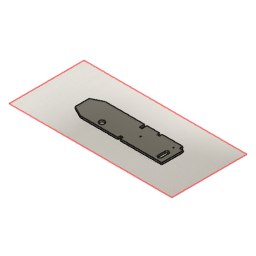
P_A22_ControlBoard v4 (Autodesk Fusion 360 design; units mm, degrees)
Autodesk Fusion 360 part; units mm, degrees
sketch "Sketch1" plane through (0, 0, 0) normal (0, 0, 1) x (1, 0, 0) in component "Component"
  line L0 (0, 23.2) -> (86.2, 23.2) construction
  line L1 (86.2, 23.2) -> (86.2, 0) construction
  line L2 (86.2, 0) -> (0, 0) construction
  line L3 (0, 0) -> (0, 23.2) construction
  line L4 (86.2, 20.3) -> (82.8, 20.3)
  line L5 (82.8, 20.3) -> (82.8, 23.2)
  line L6 (82.8, 23.2) -> (63.2045, 23.2)
  line L7 (63.3, 23.2) -> (63.3, 20.8)
  line L8 (63.3, 20.8) -> (61.1, 20.8)
  line L9 (61.1, 20.8) -> (61.1, 23.2)
  line L10 (61.1, 23.2) -> (49.1, 23.2)
  line L11 (49.1, 23.2) -> (49.1, 18.6)
  line L12 (49.1, 18.6) -> (46.9, 18.6)
  line L13 (46.9, 18.6) -> (46.9, 23.2)
  line L14 (46.9, 23.2) -> (10, 23.2)
  line L15 (10, 23.2) -> (0, 18.2)
  line L16 (0, 18.2) -> (0, 5)
  line L17 (0, 5) -> (10, 0)
  line L18 (10, 0) -> (45, 0)
  line L19 (45, 0) -> (45, 2.6)
  line L20 (45, 2.6) -> (47.2, 2.6)
  line L21 (47.2, 2.6) -> (47.2, 0)
  line L22 (47.2, 0) -> (86.2, 0)
  line L23 (86.2, 0) -> (86.2, 20.3)
  circle A0 centre (25.2, 5) radius 2.5
  line L24 (78.4, 10.9318) -> (78.4, 4.2318)
  arc A1 (78.4, 4.2318) -> (81.9, 4.2318) centre (80.15, 4.2318) ccw
  line L25 (81.9, 4.2318) -> (81.9, 10.9318)
  arc A2 (81.9, 10.9318) -> (78.4, 10.9318) centre (80.15, 10.9318) ccw
  line L26 (55.1, 12) -> (54.6, 12)
  line L27 (54.6, 12) -> (54.6, 11)
  line L28 (54.6, 11) -> (55.1, 11)
  line L29 (55.1, 11) -> (55.1, 12)
  line L30 (79, 18.2) -> (79.5, 18.2)
  line L31 (79.5, 18.2) -> (79.5, 17.7)
  line L32 (79.5, 17.7) -> (79, 17.7)
  line L33 (79, 17.7) -> (79, 18.2)
  dimension "d1" = 86.2
  dimension "d2" = 23.2
  dimension "d3" = 2.2
  dimension "d4" = 2.2
  dimension "d5" = 4.6
  dimension "d6" = 2.4
  dimension "d7" = 2.2
  dimension "d8" = 2.6
  dimension "d9" = 3.4
  dimension "d10" = 2.9
  dimension "d11" = 10
  dimension "d12" = 5
  dimension "d13" = 25.2
  dimension "d14" = 5
  dimension "d15" = 5
  dimension "d16" = 45
  dimension "d17" = 46.9
  dimension "d18" = 61.1
  dimension "d19" = 6.7
  dimension "d20" = 4.3
  dimension "d21" = 4.2318
  dimension "d22" = 1.75
  dimension "d23" = 0.5
  dimension "d24" = 55.1
  dimension "d25" = 1
  dimension "d26" = 12
  dimension "d27" = 0.5
  dimension "d28" = 0.5
  dimension "d29" = 79.5
  dimension "d30" = 5
  constraint horizontal L0
  constraint vertical L1
  constraint horizontal L2
  constraint vertical L3
  constraint coincident L2.end L3.start
  constraint coincident L1 L4.start
  constraint perpendicular L1 L4
  constraint coincident L0 L5.end
  constraint perpendicular L0 L5
  constraint coincident L0 L6.end
  constraint coincident L6 L7.start
  constraint coincident L0 L7.start
  constraint perpendicular L6 L7
  constraint perpendicular L5 L8
  constraint coincident L0 L9.end
  constraint perpendicular L0 L9
  constraint coincident L0 L10.end
  constraint perpendicular L0 L11
  constraint perpendicular L11 L12
  constraint coincident L0 L13.end
  constraint perpendicular L0 L13
  constraint coincident L0 L14.end
  constraint coincident L3 L15.end
  constraint coincident L3 L16.end
  constraint coincident L2 L17.end
  constraint coincident L2 L18.end
  constraint perpendicular L18 L19
  constraint perpendicular L19 L20
  constraint coincident L2 L21.end
  constraint perpendicular L2 L21
  constraint vertical L14.end L17.end
  constraint equal L15 L17
  constraint perpendicular L6 L24
  constraint tangent L24 A1
  constraint tangent A1 L25
  constraint perpendicular L6 L25
  constraint tangent L25 A2
  constraint tangent L24 A2
  constraint horizontal L26
  constraint vertical L27
  constraint horizontal L28
  constraint vertical L29
  constraint horizontal L30
  constraint vertical L31
  constraint horizontal L32
  constraint vertical L33
  measures "d1" distance of L0.start L0.end
  measures "d2" distance of L0 L2
  measures "d3" distance of L7.end L8.end
  measures "d4" distance of L11.end L12.end
  measures "d5" distance of L12.end L13.end
  measures "d6" distance of L8.end L9.end
  measures "d7" distance of L19.end L20.end
  measures "d8" distance of L20.end L21.end
  measures "d9" distance of L4.start L4.end
  measures "d10" distance of L4.end L5.end
  measures "d11" horizontal distance of L14.end L15.end
  measures "d12" vertical distance of L14.end L15.end
  measures "d13" distance of L3 A0.centre
  measures "d14" diameter of A0
  measures "d15" distance of L2 A0.centre
  measures "d16" distance of L16 L19
  measures "d17" distance of L13 L16
  measures "d18" distance of L9 L16
  measures "d19" distance of A1.centre A2.centre
  measures "d20" distance of L23 L25
  measures "d21" distance of L22 A1.centre
  measures "d22" radius of A2
  measures "d23" distance of L27.end L28.end
  measures "d24" distance of L16 L29
  measures "d25" distance of L26.start L28.end
  measures "d26" distance of L22 L26
  measures "d27" distance of L30.start L30.end
  measures "d28" distance of L30.start L32.end
  measures "d29" distance of L16 L31.end
  measures "d30" distance of L0 L30
extrude "Extrude1" add sketch "Sketch1" along normal blind 1.6 in component "Component"
component "Component" placed x (1, 0, 0) y (0, 1, 0) z (0, 0, 1) at (0, 0, 0)
